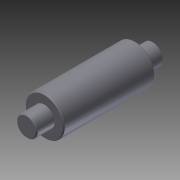
# Autodesk Inventor part: Channel - Hinge Pin
Saved by Autodesk Inventor 2011 (Build 150239000, 239)
## iProperties
Shininess: 64.0
Length Units: 11272
Angle Units: 11279
Time Units: 11290
Mass Units: 11286
Length Display Precision: 3
Angle Display Precision: 2
Compacted: True
Part Number: Channel - Hinge Pin
Document SubType Name: Modeling
Created: 2002-09-26
Designer: Autodesk, Inc.
Material: Steel, Mild
Project: Inventor Samples
Mass: 1.74089 g
Surface Area: 2.34499 cm^2
Volume: 0.221487 cm^3
Density: 7.86 g/cm^3
Density: 0.0
Volumn: 0.0
Area: 0.0
PropertySet Name: Model Information
Control State: 0
Master: False
Checked Out: False
Author: Autodesk, Inc.
Revision Number: A
Autodesk Inventor part; units mm, degrees
ref_plane "YZ Plane" through (0, 0, 0) normal (1, 0, 0) x (0, 1, 0)
ref_plane "XZ Plane" through (0, 0, 0) normal (0, 1, 0) x (-1, 0, 0)
ref_plane "XY Plane" through (0, 0, 0) normal (0, 0, 1) x (1, 0, 0)
sketch "Sketch1" plane through (0, 0, 0) normal (0, 0, 1) x (1, 0, 0)
  circle A0 centre (8.7249, -8.7376) radius 1.2573 projected
  circle A1 centre (8.7249, -8.7376) radius 2.3876
  dimension "d0" = 4.7752
  constraints: 1 centre point, 1 coincident, 1 concentric
  measures "d0" diameter of A1
extrude "Extrusion1" add sketch "Sketch1" along normal mid plane 11.176 contours A0 | A1
sketch "Sketch2" plane through (8.7249, -8.7376, 5.588) normal (0, 0, 1) x (1, 0, 0)
  circle A0 centre (0, 0) radius 1.2573 projected
extrude "Extrusion2" add sketch "Sketch2" along normal blind 2.1844
mirror "Mirror1" about plane through (0, 0, 0) normal (0, 0, 1) of "Extrusion2"
chamfer "Chamfer1" distance 0.127 angle 45 4 edges at (7.4676, -8.7376, 7.7724) (6.3373, -8.7376, 5.588) (6.3373, -8.7376, -5.588) (7.4676, -8.7376, -7.7724)
body "Solid1"
